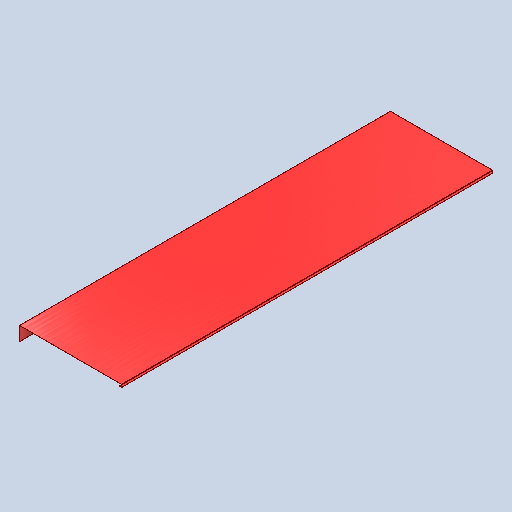
# Autodesk Inventor part: Divisor
Saved by Autodesk Inventor 2022.4 (Build 264492000, 492)
## iProperties
Created: 2022-11-09
Part Number: Divisor
Material: Generic
Document SubType Name: Sheet Metal
Designer: David
Density: 1 g/cm^3
Sheet Metal Rule: Default_mm
Appearance: Light Red
Flat Pattern Width: 42.6393 cm
Flat Pattern Length: 129.85 cm
Flat Pattern Area: 5536.71 cm^2
Sheet Metal Width: 426.393 mm
Sheet Metal Length: 1298.500 mm
Sheet Metal Area: 553671.207 mm^2
Author: David
Autodesk Inventor part; units mm, degrees
ref_plane "YZ Plane" through (0, 0, 0) normal (1, 0, 0) x (0, 1, 0)
ref_plane "XZ Plane" through (0, 0, 0) normal (0, 1, 0) x (-1, 0, 0)
ref_plane "XY Plane" through (0, 0, 0) normal (0, 0, 1) x (1, 0, 0)
sketch "Sketch2" plane through (0, 0, 0) normal (0, 1, 0) x (-1, 0, 0)
  line L0 (-179.5, 649.25) -> (179.5, 649.25)
  line L1 (179.5, 649.25) -> (179.5, -649.25)
  line L2 (179.5, -649.25) -> (-179.5, -649.25)
  line L3 (-179.5, -649.25) -> (-179.5, 649.25)
  line L4 (-179.5, 649.25) -> (179.5, -649.25) construction
  line L5 (179.5, 649.25) -> (-179.5, -649.25) construction
  point P0 (0, 0)
  dimension "d2" = 359
  dimension "d3" = 1298.5
  measures "d2" distance of L1.end L2.end
  measures "d3" distance of L0.end L1.end
extrude "Plate1" add sketch "Sketch2" along normal blind 0.5
sketch "Sketch3" plane through (-179, 0.5, -649.25) normal (-1, 0, 0) x (0, -1, 0)
  line L0 (0, 1298.5) -> (0, 0)
  line L1 (0, 0) -> (50, 0)
  line L2 (50, 0) -> (50, 1298.5)
  line L3 (50, 1298.5) -> (0, 1298.5)
  constraints: 6 end point, 1 horizontal, 1 perpendicular, 1 vertical
edge flange "Flange1" height 50 angle 90 thickness 0.5 bend radius 0.5 thickness toward (-1, 0, 0) relief straight relief width 0.5 relief depth 0.25 edges at (-179.5, 0, 0) wall of the first edge with corners at (-179, 0.5, 649.25) (-179, 0.5, -649.25) (-179, -49.5, -649.25) (-179, -49.5, 649.25)
bend "Bend1"
corner "Corner1"
sketch "Sketch6" plane through (179, 0.5, 649.25) normal (1, 0, 0) x (0, 1, 0)
  line L0 (0, -1298.5) -> (0, 0)
  line L1 (0, 0) -> (-10, 0)
  line L2 (-10, 0) -> (-10, -1298.5)
  line L3 (-10, -1298.5) -> (0, -1298.5)
  constraints: 6 end point, 1 horizontal, 1 perpendicular, 1 vertical
edge flange "Flange4" height 10 angle 90 thickness 0.5 bend radius 0.5 thickness toward (1, 0, 0) relief straight relief width 0.5 relief depth 0.25 edges at (179.5, 0, 0) wall of the first edge with corners at (179, 0.5, -649.25) (179, 0.5, 649.25) (179, -9.5, 649.25) (179, -9.5, -649.25)
bend "Bend4"
corner "Corner4"
sketch "Sketch7" plane through (179.5, -9, 649.25) normal (0, -1, 0) x (1, 0, 0)
  line L0 (0, -1298.5) -> (0, 0)
  line L1 (0, 0) -> (-10, 0)
  line L2 (-10, 0) -> (-10, -1298.5)
  line L3 (-10, -1298.5) -> (0, -1298.5)
  constraints: 6 end point, 1 horizontal, 1 perpendicular, 1 vertical
edge flange "Flange5" height 10 angle 90 thickness 0.5 bend radius 0.5 thickness toward (0, -1, 0) relief straight relief width 0.5 relief depth 0.25 edges at (179, -9.5, 0) wall of the first edge with corners at (179.5, -9, -649.25) (179.5, -9, 649.25) (169.5, -9, 649.25) (169.5, -9, -649.25)
bend "Bend5"
corner "Corner5"
equation "\"d3\" = Ancho - 3 * Thickness"
equation "\"d4\" = Thickness"
equation "\"d5\" = BendReliefWidth"
equation "\"d6\" = BendReliefDepth"
equation "\"d7\" = MinimumRemnant"
equation "\"d8\" = TransitionRadius"
equation "\"d11\" = BendRadius"
equation "\"d12\" = CornerReliefSize"
equation "\"d13\" = GapSize"
equation "\"d14\" = JacobiRadiusSize"
equation "\"d35\" = BendReliefWidth"
equation "\"d36\" = BendReliefDepth"
equation "\"d37\" = MinimumRemnant"
equation "\"d38\" = TransitionRadius"
equation "\"d41\" = BendRadius"
equation "\"d42\" = CornerReliefSize"
equation "\"d43\" = GapSize"
equation "\"d44\" = JacobiRadiusSize"
equation "\"d45\" = BendReliefWidth"
equation "\"d46\" = BendReliefDepth"
equation "\"d47\" = MinimumRemnant"
equation "\"d48\" = TransitionRadius"
equation "\"d51\" = BendRadius"
equation "\"d52\" = CornerReliefSize"
equation "\"d53\" = GapSize"
equation "\"d54\" = JacobiRadiusSize"
equation "\"BendRadius\" = Thickness"
equation "\"BendReliefWidth\" = Thickness"
equation "\"BendReliefDepth\" = 0.5 * Thickness"
equation "\"CornerReliefSize\" = 4 * Thickness"
equation "\"MinimumRemnant\" = 2 * Thickness"
equation "\"TransitionRadius\" = BendRadius"
equation "\"JacobiRadiusSize\" = BendRadius"
equation "\"GapSize\" = Thickness"
equation "\"Space7\" = 0"
equation "\"Ancho\" = 1300"
equation "\"Thickness\" = 0.5"
body "Solid1"
